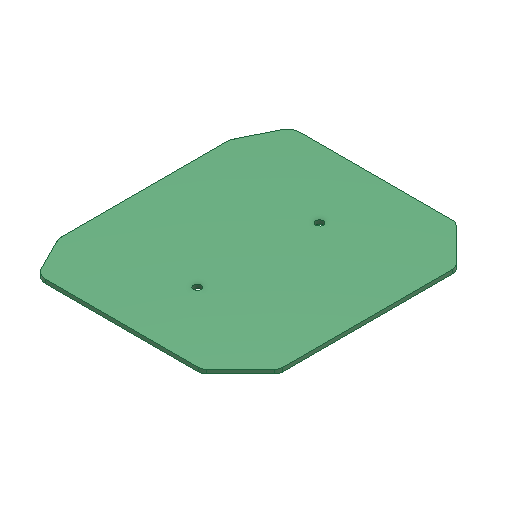
# Autodesk Inventor part: ASSEMBLY_PCB_Motherboard
Saved by Autodesk Inventor 2026.1 (Build 301233000, 233)
## iProperties
Created: 2016-05-01
Part Number: ASSEMBLY_PCB_Motherboard
Material: Ogólny
Document SubType Name: Modeling
Designer: Andrzej
Density: 1 g/cm^3
Appearance: Gładki - ciemna zieleń morska
Mass: 12.0997 g
Surface Area: 166.66 cm^2
Volume: 12.0997 cm^3
Author: Andrzej
Autodesk Inventor part; units mm, degrees
ref_plane "YZ Plane" through (0, 0, 0) normal (1, 0, 0) x (0, 1, 0)
ref_plane "XZ Plane" through (0, 0, 0) normal (0, 1, 0) x (-1, 0, 0)
ref_plane "XY Plane" through (0, 0, 0) normal (0, 0, 1) x (1, 0, 0)
sketch "Szkic1" plane through (0, 0, 0) normal (0, 0, 1) x (1, 0, 0)
  line L0 (-2.9902, 5.9208) -> (83.1098, 5.9208)
  line L1 (83.1098, 5.9208) -> (83.1098, -62.0792)
  line L2 (83.1098, -62.0792) -> (-2.9902, -62.0792)
  line L3 (-2.9902, -62.0792) -> (-2.9902, 5.9208)
  point P0 (0, 0)
  dimension "d0" = 86.1
  dimension "d1" = 68
  constraints: 8 end point, 2 parallel, 1 horizontal, 1 perpendicular
  measures "d0" distance of L1.end L2.end
  measures "d1" distance of L0.end L1.end
extrude "Wyciągnięcie proste1" add sketch "Szkic1" along normal blind 1.5
sketch "Szkic2" plane through (0, 0, 1.5) normal (0, 0, 1) x (1, 0, 0)
  point P0 (0, 0)
sketch "Szkic3" plane through (0, 0, 1.5) normal (0, 0, 1) x (1, 0, 0)
  line L0 (83.1098, 5.9208) -> (-2.9902, 5.9208) projected
  line L1 (-2.9902, 5.9208) -> (-2.9902, -62.0792) projected
  line L2 (-2.9902, -62.0792) -> (83.1098, -62.0792) projected
  line L3 (83.1098, -62.0792) -> (83.1098, 5.9208) projected
  point P0 (0, 0)
  point P1 (42.0098, -5.5792)
  point P2 (40.0098, -50.5792)
  dimension "d4" = 11.5
  dimension "d5" = 11.5
  dimension "d6" = 45
  dimension "d7" = 43
  measures "d4" distance from line of L0 point (42.01, -5.579)
  measures "d5" distance from line of L2 point (40.01, -50.579)
  measures "d6" distance from line of L1 point (42.01, -5.579)
  measures "d7" distance from line of L1 point (40.01, -50.579)
hole "Otwór1" at (42.0098, -5.5792, 1.5) at (40.0098, -50.5792, 1.5) direction (0, 0, -1) diameter 3 end through all
sketch "Szkic4" plane through (0, 0, 1.5) normal (0, 0, 1) x (1, 0, 0)
  line L0 (-2.9902, -62.0792) -> (83.1098, -62.0792) projected
  line L1 (83.1098, -62.0792) -> (83.1098, 5.9208) projected
  line L2 (83.1098, 5.9208) -> (-2.9902, 5.9208) projected
  line L3 (-2.9902, 5.9208) -> (-2.9902, -62.0792) projected
  circle A0 centre (42.0098, -5.5792) radius 1.5 projected
  circle A1 centre (40.0098, -50.5792) radius 1.5 projected
  line L4 (83.1098, 5.9208) -> (-2.9902, 5.9208) projected
  line L5 (-2.9902, 5.9208) -> (-2.9902, 20.9208)
  line L6 (-2.9902, 20.9208) -> (68.1098, 20.9208)
  line L7 (-2.9902, -62.0792) -> (-2.9902, -77.0792)
  line L8 (-2.9902, -77.0792) -> (68.1098, -77.0792)
  line L9 (-2.9902, -62.0792) -> (83.1098, -62.0792) projected
  line L10 (83.1098, -62.0792) -> (68.1098, -77.0792)
  line L11 (83.1098, -62.0792) -> (139.7388, -62.0792) construction
  line L12 (83.1098, 5.9208) -> (68.1098, 20.9208)
  line L13 (83.1098, 5.9208) -> (133.7058, 5.9208) construction
  point P0 (0, 0)
  dimension "d16" = 68
  dimension "d20" = 135
  dimension "d22" = 135
  dimension "d23" = 15
  dimension "d24" = 15
  constraints: 16 end point, 4 horizontal, 1 vertical
  measures "d16" distance of L0.end L1.end
  measures "d20" angle of L10 L11
  measures "d22" angle of L13 L12
  measures "d23" distance of L2.end L5.end
  measures "d24" distance of L0.start L7.end
extrude "Wyciągnięcie proste2" add sketch "Szkic4" against normal blind 1.5 contours L0 L10 L8 L7 | L5 L6 L12 L2
fillet "Zaokrąglenie3" radius 3 4 edges at (68.1098, -77.0792, 0.75) (83.1098, -62.0792, 0.75) (83.1098, 5.9208, 0.75) (68.1098, 20.9208, 0.75)
chamfer "Faza1" distance 8 distance2 16 1 edges at (-2.9902, -77.0792, 0.75) measured on face at (-2.4902, -77.0792, 0.75)
chamfer "Faza2" distance 8 distance2 16 1 edges at (-2.9902, 20.9208, 0.75) measured on face at (-2.4902, 20.9208, 0.75)
fillet "Zaokrąglenie4" radius 5 4 edges at (-2.9902, 4.9208, 0.75) (5.0098, 20.9208, 0.75) (5.0098, -77.0792, 0.75) (-2.9902, -61.0792, 0.75)
equation "\"d5\" = d4"
equation "\"d24\" = d23"
